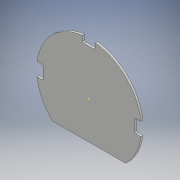
# Autodesk Inventor part: board
Saved by Autodesk Inventor 2017 (Build 210142000, 142)
## iProperties
Part Number: board
Material: Générique
Document SubType Name: Modeling
Designer: Gregwar
Density: 1 g/cm^3
Appearance: Par défaut
Author: Gregwar
Autodesk Inventor part; units mm, degrees
ref_plane "YZ Plane" through (0, 0, 0) normal (1, 0, 0) x (0, 1, 0)
ref_plane "XZ Plane" through (0, 0, 0) normal (0, 1, 0) x (-1, 0, 0)
ref_plane "XY Plane" through (0, 0, 0) normal (0, 0, 1) x (1, 0, 0)
sketch "Esquisse1" plane through (0, 0, 0) normal (0, 1, 0) x (-1, 0, 0)
  circle A0 centre (0, 0) radius 80
  dimension "d0" = 160
  constraints: 1 centre point, 1 coincident
  measures "d0" diameter of A0
extrude "Extrusion1" add sketch "Esquisse1" along normal blind 3
sketch "Esquisse2" plane through (0, 3, 0) normal (0, 1, 0) x (1, 0, 0)
  line L0 (-80, -10) -> (-70, -10)
  line L1 (-70, -10) -> (-70, 10)
  line L2 (-70, 10) -> (-80, 10)
  line L3 (-80, 10) -> (-80, -10)
  line L4 (0, 0) -> (-70, 0) construction
  line L5 (0, 0) -> (0, 254.2105) construction
  line L6 (10, -80) -> (10, -70)
  line L7 (10, -70) -> (-10, -70)
  line L8 (-10, -70) -> (-10, -80)
  line L9 (-10, -80) -> (10, -80)
  line L10 (80, 10) -> (70, 10)
  line L11 (70, 10) -> (70, -10)
  line L12 (70, -10) -> (80, -10)
  line L13 (80, -10) -> (80, 10)
  point P0 (0, -70)
  point P1 (70, 0)
  dimension "d3" = 20
  dimension "d5" = 80
  dimension "d6" = 10
  dimension "d9" = 180
  constraints: 28 end point, 2 parallel, 2 perpendicular, 1 horizontal, 1 midpoint, 1 vertical, 19 other
  measures "d3" distance of L2.end L0.start
  measures "d5" distance between parallel lines of L3 L5
  measures "d6" distance of L1.end L2.end
extrude "Extrusion2" cut sketch "Esquisse2" against normal through all
fillet "Congé1" radius 2 6 edges at (-70, 1.5, -10) (-70, 1.5, 10) (70, 1.5, -10) (70, 1.5, 10) (10, 1.5, 70) (-10, 1.5, 70)
sketch "Esquisse4" plane through (0, 0, 0) normal (0, -1, 0) x (1, 0, 0)
  point P0 (0, 0)
sketch "Esquisse5" plane through (0, 3, 0) normal (0, 1, 0) x (1, 0, 0)
  line L0 (-100, 57) -> (100, 57)
  line L1 (100, 57) -> (100, 80)
  line L2 (100, 80) -> (-100, 80)
  line L3 (-100, 80) -> (-100, 57)
  line L4 (-10, -79.3725) -> (-10, -72) construction
  arc A0 (-8, -70) -> (-10, -72) centre (-8, -72) ccw construction
  line L5 (-8, -70) -> (8, -70) construction
  arc A1 (10, -72) -> (8, -70) centre (8, -72) ccw construction
  line L6 (10, -72) -> (10, -79.3725) construction
  arc A2 (10, -79.3725) -> (79.3725, -10) centre (0, 0) ccw construction
  line L7 (79.3725, -10) -> (72, -10) construction
  arc A3 (70, -8) -> (72, -10) centre (72, -8) ccw construction
  line L8 (70, -8) -> (70, 8) construction
  arc A4 (72, 10) -> (70, 8) centre (72, 8) ccw construction
  line L9 (72, 10) -> (79.3725, 10) construction
  arc A5 (79.3725, 10) -> (-79.3725, 10) centre (0, 0) ccw construction
  line L10 (-79.3725, 10) -> (-72, 10) construction
  arc A6 (-70, 8) -> (-72, 10) centre (-72, 8) ccw construction
  line L11 (-70, 8) -> (-70, -8) construction
  arc A7 (-72, -10) -> (-70, -8) centre (-72, -8) ccw construction
  line L12 (-72, -10) -> (-79.3725, -10) construction
  arc A8 (-79.3725, -10) -> (-10, -79.3725) centre (0, 0) ccw construction
  line L13 (0, 0) -> (0, 237.415) construction
  point P0 (0, 80)
  dimension "d17" = 200
  dimension "d18" = 23
  constraints: 10 end point, 2 parallel, 1 horizontal, 1 midpoint, 1 perpendicular, 1 point on circle, 1 point on line, 1 vertical
  measures "d17" distance of L0.start L0.end
  measures "d18" distance between parallel lines of L2 L0
extrude "Extrusion4" cut sketch "Esquisse5" against normal through all
